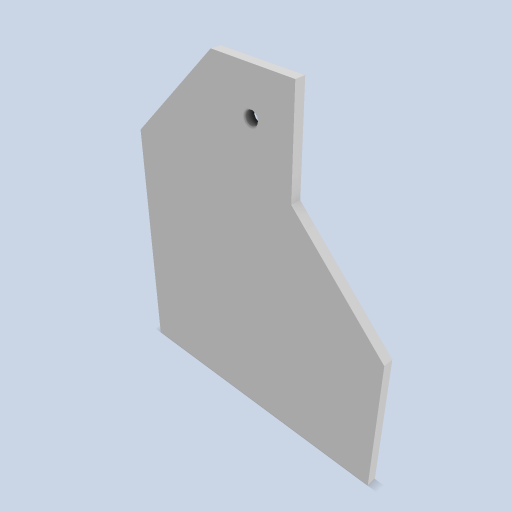
# Autodesk Inventor part: base side
Saved by Autodesk Inventor 2023 (Build 270158000, 158)
## iProperties
Created: 2022-10-13
Part Number: base side
Material: Generic
Document SubType Name: Modeling
Designer: Nathan
Density: 1 g/cm^3
Appearance: Default
Author: Nathan
Autodesk Inventor part; units mm, degrees
ref_plane "YZ Plane" through (0, 0, 0) normal (1, 0, 0) x (0, 1, 0)
ref_plane "XZ Plane" through (0, 0, 0) normal (0, 1, 0) x (-1, 0, 0)
ref_plane "XY Plane" through (0, 0, 0) normal (0, 0, 1) x (1, 0, 0)
sketch "Sketch1" plane through (0, 0, 0) normal (0, 0, 1) x (1, 0, 0)
  line L0 (0, 0) -> (508, 0)
  line L1 (508, 0) -> (508, 609.6)
  line L2 (508, 609.6) -> (0, 609.6)
  line L3 (0, 609.6) -> (0, 0)
  line L4 (254, 609.6) -> (177.8, 609.6)
  line L5 (177.8, 609.6) -> (125.7631, 609.6)
  line L6 (254, 609.6) -> (330.2, 609.6)
  line L7 (177.8, 609.6) -> (0, 431.8)
  line L8 (177.8, 609.6) -> (429.2472, 609.6) construction
  line L9 (330.2, 609.6) -> (330.2, 431.8)
  line L10 (330.2, 431.8) -> (508, 254)
  circle A0 centre (254, 533.4) radius 12.7
  dimension "d0" = 508
  dimension "d1" = 609.6
  dimension "d2" = 76.2
  dimension "d3" = 76.2
  dimension "d4" = 135
  dimension "d5" = 135
  dimension "d6" = 25.4
  dimension "d7" = 76.2
  dimension "d10" = 177.8
  dimension "d11" = 538.8154
  dimension "d12" = 254
  dimension "d13" = 382.2369
  dimension "d14" = 254
  constraints: 22 end point, 5 point on line, 2 horizontal, 2 parallel, 1 centre point, 1 equal length, 1 midpoint, 1 perpendicular, 1 vertical
  measures "d0" distance of L2.end L1.end
  measures "d1" distance of L1.end L0.end
  measures "d2" distance of L4.start L4.end
  measures "d3" distance of L4.start L6.end
  measures "d4" angle of L7 L8
  measures "d5" angle of L10 L9
  measures "d6" diameter of A0
  measures "d7" distance of A0.centre L4.start
  measures "d10" horizontal distance of L7.end L4.end
  measures "d11" distance from line of L0.start L10
  measures "d12" distance from line of A0.centre L1
  measures "d13" distance from line of L5.end L1
  measures "d14" distance of L0.end L10.end
extrude "Extrusion1" add sketch "Sketch1" along normal blind 18.0086 contours L3 L7 L2 L9 L10 L1 L0
body "Solid1"
